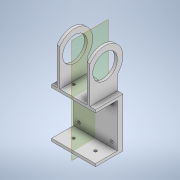
# Autodesk Inventor part: Intake - Mount
Saved by Autodesk Inventor 2020 (Build 240168000, 168)
## iProperties
Created: 2020-02-05
Part Number: Intake - Mount
Material: Generic
Document SubType Name: Modeling
Designer: aidan
Density: 1 g/cm^3
Appearance: Default
Author: aidan
Autodesk Inventor part; units mm, degrees
ref_plane "YZ Plane" through (0, 0, 0) normal (1, 0, 0) x (0, 1, 0)
ref_plane "XZ Plane" through (0, 0, 0) normal (0, 1, 0) x (-1, 0, 0)
ref_plane "XY Plane" through (0, 0, 0) normal (0, 0, 1) x (1, 0, 0)
sketch "Sketch1" plane through (0, 0, 0) normal (0, 1, 0) x (-1, 0, 0)
  line L0 (0, 0) -> (-50.8, 0)
  line L1 (-50.8, 0) -> (-50.8, -25.4)
  line L2 (-50.8, -25.4) -> (0, -25.4)
  line L3 (0, -25.4) -> (0, 0)
  dimension "d0" = 50.8
  dimension "d1" = 25.4
  constraints: 8 end point, 2 parallel, 1 horizontal, 1 perpendicular
  measures "d0" distance of L2.end L1.end
  measures "d1" distance of L1.end L0.end
extrude "Extrusion1" add sketch "Sketch1" along normal blind 3.175
sketch "Sketch10" plane through (0, 3.175, 0) normal (0, 1, 0) x (1, 0, 0)
  line L0 (50.8, 25.4) -> (0, 25.4) projected
  line L1 (0, 25.4) -> (50.8, 25.4)
  line L2 (50.8, 25.4) -> (50.8, 31.75)
  line L3 (50.8, 31.75) -> (0, 31.75)
  line L4 (0, 31.75) -> (0, 25.4)
  point P0 (0, 0)
  dimension "d46" = 6.35
  constraints: 8 end point, 2 parallel, 1 horizontal, 1 perpendicular
  measures "d46" distance of L1.end L2.end
extrude "Extrusion7" add sketch "Sketch10" against normal blind 57.15
sketch "Sketch11" plane through (50.8, 0, 0) normal (1, 0, 0) x (0, 0, -1)
  line L0 (25.4, -53.975) -> (31.75, -53.975) projected
  line L1 (25.4, -53.975) -> (0, -53.975)
  line L2 (0, -53.975) -> (0, -50.8)
  line L3 (0, -50.8) -> (25.4, -50.8)
  line L4 (25.4, -50.8) -> (25.4, -53.975)
  point P0 (0, 0)
  dimension "d49" = 3.175
  dimension "d80" = 25.4
  constraints: 8 end point, 2 parallel, 1 horizontal, 1 perpendicular
  measures "d49" distance of L1.end L2.end
  measures "d80" distance of L2.end L3.end
extrude "Extrusion8" add sketch "Sketch11" against normal blind 50.8
sketch "Sketch12" plane through (0, 3.175, 0) normal (0, 1, 0) x (1, 0, 0)
  line L0 (6.35, 31.75) -> (9.525, 31.75)
  line L1 (9.525, 31.75) -> (9.525, 0)
  line L2 (9.525, 0) -> (6.35, 0)
  line L3 (6.35, 0) -> (6.35, 31.75)
  line L4 (41.275, 31.75) -> (44.45, 31.75)
  line L5 (44.45, 31.75) -> (44.45, 0)
  line L6 (44.45, 0) -> (41.275, 0)
  line L7 (41.275, 0) -> (41.275, 31.75)
  line L8 (9.525, 31.75) -> (41.275, 31.75) construction
  line L9 (50.8, 25.4) -> (0, 25.4) construction
  line L10 (50.8, 31.75) -> (0, 31.75) construction
  line L11 (50.8, 0) -> (50.8, 31.75) construction
  point P0 (0, 0)
  point P1 (25.4, 31.75)
  point P2 (25.4, 31.75)
  point P3 (44.45, 15.875)
  point P4 (50.8, 15.875)
  point P5 (42.8625, 31.75)
  point P6 (25.4, 31.75)
  dimension "d52" = 31.75
  dimension "d54" = 3.175
  constraints: 18 end point, 6 midpoint, 5 parallel, 2 horizontal, 2 horizontal alignment, 2 perpendicular, 2 point on line, 1 coincident, 1 collinear
  measures "d52" distance between parallel lines of L7 L1
  measures "d54" distance of L0.start L0.end
extrude "Extrusion9" add sketch "Sketch12" along normal blind 76.2
sketch "Sketch14" plane through (0, 3.175, 0) normal (0, 1, 0) x (1, 0, 0)
  line L0 (0, 31.75) -> (0, 0) projected
  line L1 (0, 0) -> (50.8, 0) projected
  point P0 (12.7, 12.7)
  point P1 (38.1, 12.7)
  dimension "d62" = 12.7
  dimension "d63" = 12.7
  dimension "d64" = 25.4
  constraints: 1 horizontal alignment
  measures "d62" distance from line of L0 point (12.7, 12.7)
  measures "d63" distance from line of L1 point (12.7, 12.7)
  measures "d64" distance of point (12.7, 12.7) point (38.1, 12.7)
hole "Hole3" at (12.7, 3.175, -12.7) at (38.1, 3.175, -12.7) direction (0, -1, 0) diameter 3.175 end through all
sketch "Sketch15" plane through (50.8, 3.175, -31.75) normal (0, 0, -1) x (-1, 0, 0)
  line L0 (6.35, -9.525) -> (44.45, -9.525) construction
  line L1 (44.45, -9.525) -> (44.45, -47.625) construction
  line L2 (44.45, -47.625) -> (6.35, -47.625) construction
  line L3 (6.35, -47.625) -> (6.35, -9.525) construction
  line L4 (0, 0) -> (50.8, 0) construction
  line L5 (50.8, 0) -> (50.8, -57.15) construction
  point P0 (50.8, -3.175)
  point P1 (25.4, -9.525)
  point P2 (25.4, 0)
  point P3 (44.45, -28.575)
  point P4 (50.8, -28.575)
  dimension "d72" = 38.1
  constraints: 8 end point, 4 midpoint, 2 parallel, 2 perpendicular, 1 horizontal, 1 horizontal alignment, 1 vertical alignment
  measures "d72" distance of L0.start L0.end
hole "Hole4" at (44.45, -6.35, -31.75) at (6.35, -6.35, -31.75) at (6.35, -44.45, -31.75) at (44.45, -44.45, -31.75) direction (0, 0, 1) diameter 3.175 end through all
sketch "Sketch17" plane through (6.35, 3.175, -31.75) normal (-1, 0, 0) x (0, 0, 1)
  circle A0 centre (14.2875, 31.75) radius 14.2875
  line L0 (0, 0) -> (31.75, 0) projected
  line L1 (31.75, 0) -> (31.75, 76.2) projected
  line L2 (0, 76.2) -> (31.75, 76.2) projected
  line L3 (31.75, 76.2) -> (0, 76.2)
  line L4 (0, 76.2) -> (0, 33.9421)
  line L5 (0, 0) -> (0, 76.2) projected
  arc A1 (31.75, 42.7485) -> (31.75, 20.7515) centre (14.2875, 31.75) ccw
  point P0 (31.75, -3.175)
  point P1 (31.75, 30.0485)
  point P2 (0, 46.6421)
  point P3 (0, 16.8579)
  dimension "d83" = 28.575
  dimension "d84" = 31.75
  dimension "d85" = 17.4625
  dimension "d98" = 6.35
  constraints: 4 end point, 4 point on line, 2 centre point, 2 point on circle, 1 collinear
  measures "d83" diameter of A0
  measures "d84" distance from line of L0 A0.centre
  measures "d85" distance from line of L1 A0.centre
  measures "d98" radial gap between concentric circles of A0 A1
extrude "Extrusion16" cut sketch "Sketch17" against normal blind 38.1 contours A0 | L4 L2 L1 A1
extrude "Extrusion17" add sketch "Sketch17" against normal blind 3.175 contours L5 A1 L4
ref_plane "Work Plane2" through (25.4, 3.175, -31.75) normal (-1, 0, 0) x (0, 0, 1)
mirror "Mirror2" about plane through (25.4, 3.175, -31.75) normal (-1, 0, 0) of "Extrusion17"
body "Solid1"
